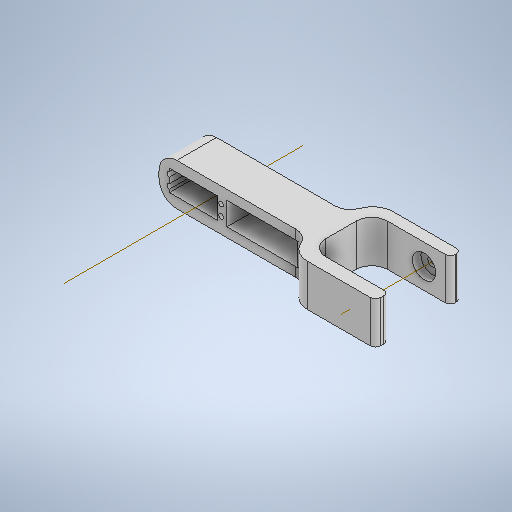
# Autodesk Inventor part: inferior arm
Saved by Autodesk Inventor 2025 (Build 290162000, 162)
## iProperties
Created: 2024-11-29
Part Number: inferior arm
Material: Generic
Document SubType Name: Modeling
Designer: Pauline Simonnet
Density: 1 g/cm^3
Appearance: Default
Author: Pauline Simonnet
Autodesk Inventor part; units mm, degrees
ref_plane "YZ Plane" through (0, 0, 0) normal (1, 0, 0) x (0, 1, 0)
ref_plane "XZ Plane" through (0, 0, 0) normal (0, 1, 0) x (-1, 0, 0)
ref_plane "XY Plane" through (0, 0, 0) normal (0, 0, 1) x (1, 0, 0)
sketch "Sketch1" plane through (0, 0, 0) normal (0, 1, 0) x (-1, 0, 0)
  line L0 (0, 0) -> (65, 0)
  line L1 (65, 0) -> (65, -38)
  line L2 (65, -38) -> (0, -38)
  line L3 (0, -38) -> (0, 0)
  dimension "d0" = 38
  dimension "d1" = 65
  constraints: 8 end point, 2 parallel, 1 horizontal, 1 perpendicular
  measures "d0" distance between parallel lines of L2 L0
  measures "d1" distance of L1.end L2.end
extrude "Extrusion1" add sketch "Sketch1" along normal blind 40
sketch "Sketch2" plane through (-65, 0, 0) normal (0, 0, 1) x (1, 0, 0)
  line L0 (10, 30.15) -> (56, 30.15)
  line L1 (56, 30.15) -> (56, 9.85)
  line L2 (56, 9.85) -> (10, 9.85)
  line L3 (10, 9.85) -> (10, 30.15)
  line L4 (0, 40) -> (65, 40) projected
  line L5 (0, 0) -> (0, 40) projected
  line L6 (65, 0) -> (65, 40) projected
  dimension "d4" = 46
  dimension "d5" = 20.3
  dimension "d6" = 9.85
  dimension "d19" = 10
  constraints: 8 end point, 2 parallel, 1 horizontal, 1 perpendicular
  measures "d4" distance of L0.start L0.end
  measures "d5" distance of L0.end L1.end
  measures "d6" distance between parallel lines of L0 L4
  measures "d19" distance between parallel lines of L3 L5
extrude "Extrusion2" cut sketch "Sketch2" against normal blind 35
sketch "Sketch5" plane through (-65, 0, -35) normal (0, 0, 1) x (1, 0, 0)
  circle A0 centre (45, 20) radius 4.5
  line L0 (10, 30.15) -> (56, 30.15) projected
  line L1 (10, 9.85) -> (10, 30.15) projected
  line L2 (56, 30.15) -> (56, 9.85) projected
  point P0 (65, 0)
  dimension "d20" = 9
  dimension "d21" = 10.15
  dimension "d45" = 11
  constraints: 1 centre point
  measures "d20" diameter of A0
  measures "d21" distance from line of L0 A0.centre
  measures "d45" distance from line of L2 A0.centre
extrude "Extrusion5" cut sketch "Sketch5" against normal through all
sketch "Sketch6" plane through (0, 0, 0) normal (0, -1, 0) x (1, 0, 0)
  line L0 (-65, -38) -> (75, -38)
  line L1 (75, -38) -> (75, 0)
  line L2 (75, 0) -> (-65, 0)
  line L3 (-65, 0) -> (-65, -38)
  line L4 (0, 0) -> (0, -38) projected
  line L5 (-65, 0) -> (0, 0) projected
  dimension "d27" = 75
  dimension "d34" = 0
  constraints: 8 end point, 2 parallel, 1 horizontal, 1 perpendicular
  measures "d27" distance between parallel lines of L1 L4
  measures "d34" distance between parallel lines of L2 L5
extrude "Extrusion6" add sketch "Sketch6" against normal blind 9
sketch "Sketch7" plane through (0, 40, 0) normal (0, 1, 0) x (1, 0, 0)
  line L0 (-65, 0) -> (0, 0) projected
  line L1 (0, 38) -> (75, 38) projected
  line L2 (-65, 0) -> (75, 0)
  line L3 (75, 0) -> (75, 38)
  line L4 (75, 38) -> (-65, 38)
  line L5 (-65, 38) -> (-65, 0)
  constraints: 8 end point, 2 parallel, 1 horizontal, 1 perpendicular
extrude "Extrusion7" add sketch "Sketch7" against normal blind 9
sketch "Sketch8" plane through (-9, 9.85, 0) normal (-1, 0, 0) x (0, 0, 1)
  line L0 (-29, 5.15) -> (-19, 5.15)
  line L1 (-19, 5.15) -> (-19, 15.15)
  line L2 (-19, 15.15) -> (-29, 15.15)
  line L3 (-29, 15.15) -> (-29, 5.15)
  line L4 (-35, 20.3) -> (-35, 0) projected
  line L5 (0, 0) -> (-35, 0) projected
  line L6 (0, 20.3) -> (0, 0) projected
  point P0 (0, -9.85)
  point P1 (-35, 0.15)
  point P2 (0, 0.15)
  point P3 (-35, 20.15)
  point P4 (0, 20.15)
  dimension "d36" = 10
  dimension "d37" = 10
  dimension "d39" = 5.15
  dimension "d42" = 19
  constraints: 8 end point, 2 parallel, 1 horizontal, 1 perpendicular
  measures "d36" distance between parallel lines of L1 L3
  measures "d37" distance between parallel lines of L2 L0
  measures "d39" distance between parallel lines of L0 L5
  measures "d42" distance between parallel lines of L1 L6
extrude "Extrusion8" cut sketch "Sketch8" against normal blind 28
sketch "Sketch10" plane through (75, 0, 0) normal (1, 0, 0) x (0, 0, 1)
  line L0 (0, -9) -> (-38, -9)
  line L1 (-38, -9) -> (-38, -31)
  line L2 (-38, -31) -> (0, -31)
  line L3 (0, -31) -> (0, -9)
  point P0 (0, 0)
  constraints: 8 end point, 2 parallel, 1 horizontal, 1 perpendicular
extrude "Extrusion10" add sketch "Sketch10" against normal blind 2
sketch "Sketch11" plane through (73, 0, 0) normal (-1, 0, 0) x (0, 0, 1)
  line L0 (-38, 40) -> (0, 40)
  line L1 (0, 40) -> (0, 0)
  line L2 (0, 0) -> (-38, 0)
  line L3 (-38, 0) -> (-38, 40)
  line L4 (-38, 31) -> (-38, 9) projected
  point P0 (0, 0)
  point P1 (-38, 40)
  constraints: 8 end point, 2 coincident, 2 parallel, 1 horizontal, 1 perpendicular
extrude "Extrusion11" add sketch "Sketch11" along normal mid plane 10
sketch "Sketch17" plane through (0, 0, 0) normal (0, 0, 1) x (1, 0, 0)
  circle A0 centre (-5.6, 15) radius 2.25
  circle A1 centre (-5.6, 25) radius 2.25
  circle A2 centre (-55, 15) radius 2.25
  circle A3 centre (-55, 25) radius 2.25
  line L0 (-9, 30.15) -> (-9, 9.85) projected
  line L1 (-55, 30.15) -> (-9, 30.15) projected
  line L2 (-55, 9.85) -> (-55, 30.15) projected
  point P0 (0, 0)
  point P1 (-9, 10)
  point P2 (-55, 10)
  point P3 (-9, 30)
  point P4 (-55, 30)
  dimension "d105" = 4.5
  dimension "d107" = 10
  dimension "d108" = 10
  dimension "d109" = 3.4
  dimension "d110" = 3.4
  dimension "d111" = 5.15
  dimension "d112" = 5.15
  dimension "d113" = 0
  dimension "d114" = 0
  constraints: 4 centre point, 3 equal radius
  measures "d105" diameter of A3
  measures "d107" distance of A3.centre A2.centre
  measures "d108" distance of A1.centre A0.centre
  measures "d109" distance from line of L0 A1.centre
  measures "d110" distance from line of L0 A0.centre
  measures "d111" distance from line of L1 A1.centre
  measures "d112" distance from line of L1 A3.centre
  measures "d113" distance from line of L2 A2.centre
  measures "d114" distance from line of L2 A3.centre
extrude "Extrusion17" cut sketch "Sketch17" against normal blind 20
sketch "Sketch18" plane through (0, 0, 0) normal (0, -1, 0) x (1, 0, 0)
  line L0 (78, -54) -> (163, -54)
  line L1 (163, -54) -> (163, 16)
  line L2 (163, 16) -> (78, 16)
  line L3 (78, 16) -> (78, -54)
  line L4 (78, 0) -> (78, -38) projected
  line L5 (78, -38) -> (-65, -38) projected
  point P0 (0, 0)
  dimension "d118" = 85
  dimension "d119" = 70
  dimension "d120" = 0
  dimension "d121" = 16
  constraints: 8 end point, 2 parallel, 1 horizontal, 1 perpendicular
  measures "d118" distance of L1.end L2.end
  measures "d119" distance between parallel lines of L2 L0
  measures "d120" distance between parallel lines of L3 L4
  measures "d121" distance between parallel lines of L5 L0
extrude "Extrusion18" add sketch "Sketch18" against normal blind 40
sketch "Sketch19" plane through (0, 0, 0) normal (0, -1, 0) x (1, 0, 0)
  line L0 (163, 16) -> (163, -54) projected
  line L1 (163, -50.5) -> (88, -50.5)
  line L2 (88, -50.5) -> (88, 8.5)
  line L3 (88, 8.5) -> (163, 8.5)
  line L4 (163, 8.5) -> (163, -50.5)
  line L5 (163, 16) -> (78, 16) projected
  point P0 (0, 0)
  dimension "d124" = 75
  dimension "d125" = 59
  dimension "d126" = 7.5
  constraints: 8 end point, 2 parallel, 1 horizontal, 1 perpendicular, 1 point on line
  measures "d124" distance of L1.start L1.end
  measures "d125" distance of L1.end L2.end
  measures "d126" distance between parallel lines of L5 L3
extrude "Extrusion19" cut sketch "Sketch19" against normal blind 40
sketch "Sketch20" plane through (163, 0, 8.5) normal (0, 0, -1) x (-1, 0, 0)
  circle A0 centre (25, 20) radius 4.25
  line L0 (0, 0) -> (0, 40) projected
  line L1 (0, 40) -> (85, 40) projected
  point P0 (163, 0)
  dimension "d129" = 8.5
  dimension "d130" = 25
  dimension "d131" = 20
  constraints: 1 centre point
  measures "d129" diameter of A0
  measures "d130" distance from line of L0 A0.centre
  measures "d131" distance from line of A0.centre L1
extrude "Extrusion20" cut sketch "Sketch20" against normal blind 40
sketch "Sketch21" plane through (163, 0, -54) normal (0, 0, -1) x (-1, 0, 0)
  line L0 (85, 0) -> (85, 40) projected
  line L1 (85, 40) -> (0, 40)
  line L2 (0, 40) -> (0, 0)
  line L3 (0, 0) -> (85, 0)
  line L4 (85, 0) -> (85, 40)
  line L5 (85, 0) -> (0, 0) projected
  point P0 (163, 0)
  constraints: 8 end point, 2 parallel, 2 perpendicular, 1 horizontal
extrude "Extrusion21" add sketch "Sketch21" along normal blind 7
sketch "Sketch22" plane through (78, 0, 16) normal (0, 0, 1) x (1, 0, 0)
  line L0 (10, 40) -> (85, 40) projected
  line L1 (0, 0) -> (85, 0)
  line L2 (85, 0) -> (85, 40)
  line L3 (85, 40) -> (0, 40)
  line L4 (0, 40) -> (0, 0)
  line L5 (85, 0) -> (0, 0) projected
  constraints: 8 end point, 2 parallel, 2 perpendicular, 1 horizontal
extrude "Extrusion22" add sketch "Sketch22" along normal blind 5
sketch "Sketch23" plane through (138, 20, 16) normal (0, 0, -1) x (-1, 0, 0)
  line L0 (10.8, 3.875) -> (0, 6.8)
  line L1 (10.8, -3.875) -> (0, -6.8)
  circle A0 centre (10.8, 0) radius 1.5
  line L2 (0, 0) -> (21.6, 0) construction
  line L3 (10.8, 3.875) -> (17.8, 3.875)
  line L4 (10.8, 0) -> (10.8, 7.3195) construction
  line L5 (10.8, -3.875) -> (17.8, -3.875)
  circle A1 centre (17.8, 0) radius 1.5
  arc A2 (17.8, -3.875) -> (17.8, 3.875) centre (17.8, 0) ccw
  circle A3 centre (0, 0) radius 2.75
  arc A4 (0, 6.8) -> (0, -6.8) centre (0, 0) ccw
  circle A5 centre (0, 0) radius 4.25
  circle A6 centre (0, 0) radius 4.25 projected
  point P0 (138, -20)
  point P1 (-3.1396, 10.9667)
  dimension "d138" = 13.6
  dimension "d139" = 7.75
  dimension "d140" = 17.8
  dimension "d141" = 0
  dimension "d142" = 5.5
  dimension "d143" = 3
  dimension "d144" = 3
  dimension "d145" = 7
  dimension "d146" = 17.8
  dimension "d147" = 0
  dimension "d148" = 0
  dimension "d149" = 0
  dimension "d150" = 0
  dimension "d151" = 7.75
  dimension "d152" = 0
  dimension "d153" = 0
  constraints: 12 end point, 6 centre point, 4 point on circle, 3 horizontal, 2 coincident, 1 midpoint, 1 point on line, 1 vertical
  measures "d138" diameter of A4
  measures "d139" diameter of A2
  measures "d140" distance of point (0, 0) A2.centre
  measures "d141" distance from line of L2 A2.centre
  measures "d142" diameter of A3
  measures "d143" diameter of A0
  measures "d144" diameter of A1
  measures "d145" distance of L4.start A1.centre
  measures "d146" distance of point (0, 0) A1.centre
  measures "d147" distance from line of L4 L1.start
  measures "d148" distance from line of L4 L0.start
  measures "d149" distance of A3.centre A5.centre
  measures "d150" distance of L2.start A5.centre
  measures "d151" distance between parallel lines of L5 L3
  measures "d152" distance of A6.centre point (0, 0)
  measures "d153" distance of A6.centre L2.start
extrude "Extrusion23" cut sketch "Sketch23" along normal blind 9 contours L3 A2 L5 L1 A4 L0 | A0 | A1 | A3 | A5
sketch "Sketch24" plane through (163, 0, -61) normal (0, 0, -1) x (-1, 0, 0)
  arc A0 (25, 26.8) -> (25, 13.2) centre (25, 20) ccw projected
  circle A1 centre (25, 20) radius 4.5
  point P0 (163, 0)
  dimension "d156" = 9
  constraints: 1 centre point, 1 coincident
  measures "d156" diameter of A1
extrude "Extrusion24" cut sketch "Sketch24" against normal blind 13
sketch "Sketch25" plane through (88, 0, -50.5) normal (0, 0, 1) x (1, 0, 0)
  circle A0 centre (50, 20) radius 4.5 projected
  circle A1 centre (50, 20) radius 11.14
  point P0 (-88, 0)
  dimension "d159" = 22.28
  constraints: 1 centre point, 1 coincident
  measures "d159" diameter of A1
extrude "Extrusion25" cut sketch "Sketch25" against normal blind 8
fillet "Fillet10" radius 20 2 edges at (78, 20, 21) (78, 20, -61)
fillet "Fillet11" radius 15 2 edges at (88, 20, 8.5) (88, 20, -50.5)
fillet "Fillet12" radius 15 2 edges at (78, 20, -38) (78, 20, 0)
fillet "Fillet13" radius 5 4 edges at (163, 20, 21) (163, 20, 8.5) (163, 20, -50.5) (163, 20, -61)
fillet "Fillet14" radius 17 2 edges at (-65, 0, -19) (-65, 40, -19)
equation "\"d110\" = d109"
equation "\"d112\" = d111"
body "Solid1"
